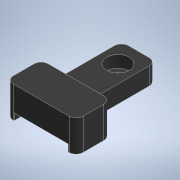
# Autodesk Inventor part: 28_Switch_Holder_Y
Saved by Autodesk Inventor 2022.2 (Build 262287010, 287A)
## iProperties
Created: 2022-05-06
Part Number: 28_Switch_Holder_Y
Material: PET-Kunststoff
Document SubType Name: Modeling
Designer: MXBD
Density: 1.541 g/cm^3
Appearance: Gummi - Schwarz
Author: MXBD
Autodesk Inventor part; units mm, degrees
ref_plane "YZ Plane" through (0, 0, 0) normal (1, 0, 0) x (0, 1, 0)
ref_plane "XZ Plane" through (0, 0, 0) normal (0, 1, 0) x (-1, 0, 0)
ref_plane "XY Plane" through (0, 0, 0) normal (0, 0, 1) x (1, 0, 0)
sketch "Skizze1" plane through (0, 0, 0) normal (0, 1, 0) x (-1, 0, 0)
  line L0 (0, -28.6) -> (0, 10.6) projected
  line L1 (-14, 0) -> (14, 0) projected
  line L2 (-10, 5) -> (10, 5)
  line L3 (10, 5) -> (10, -5)
  line L4 (10, -5) -> (-10, -5)
  line L5 (-10, -5) -> (-10, 5)
  line L6 (-10, 5) -> (10, -5) construction
  line L7 (10, 5) -> (-10, -5) construction
  line L8 (-5, -5) -> (5, -5)
  line L9 (5, -5) -> (5, -23)
  line L10 (5, -23) -> (-5, -23)
  line L11 (-5, -23) -> (-5, -5)
  line L12 (-5, -5) -> (5, -23) construction
  line L13 (5, -5) -> (-5, -23) construction
  point P0 (0, 0)
  point P1 (0, -14)
  point P2 (-5, -5)
  point P3 (5, -5)
  dimension "d0" = 20
  dimension "d1" = 10
  dimension "d2" = 10
  dimension "d3" = 18
  constraints: 24 end point, 4 midpoint, 4 parallel, 2 horizontal, 2 perpendicular, 1 collinear, 1 point on line
  measures "d0" distance of L3.end L4.end
  measures "d1" distance of L2.end L3.end
  measures "d2" distance of L9.end L10.end
  measures "d3" distance of L8.end L9.end
extrude "Extrusion1" add sketch "Skizze1" along normal blind 5
sketch "Skizze2" plane through (0, 5, 0) normal (0, 1, 0) x (1, 0, 0)
  line L0 (0, 28.6) -> (0, -10.6) projected
  line L1 (5, 23) -> (-5, 23) projected
  line L2 (-10, -5) -> (10, -5) projected
  point P0 (0, 0)
  point P1 (0, 17)
  dimension "d14" = 22
  constraints: 1 point on line
  measures "d14" distance from line of point (0, 17) L2
hole "Bohrung1" at (0, 5, -17) direction (0, -1, 0) diameter 3.4 end through all counterbore diameter 6.5 counterbore depth 3.4 clearance for "Inbusschraube ISO 4762" size "M3" standard "ISO"
sketch "Skizze3" plane through (0, 5, 0) normal (0, 1, 0) x (1, 0, 0)
  line L0 (-10, -5) -> (10, -5) projected
  line L1 (10, -5) -> (10, 5) projected
  line L2 (-10, -5) -> (10, -5)
  line L3 (10, -5) -> (10, 5)
  line L4 (10, 5) -> (-10, 5)
  line L5 (-10, 5) -> (-10, -5)
  point P0 (0, 0)
  constraints: 8 end point, 2 parallel, 1 horizontal, 1 perpendicular
extrude "Extrusion2" add sketch "Skizze3" along normal blind 2
sketch "Skizze4" plane through (0, 0, 0) normal (0, -1, 0) x (1, 0, 0)
  line L0 (-10, 5) -> (10, 5) projected
  line L1 (10, -5) -> (5, -5) projected
  line L2 (10, 5) -> (7.75, 5)
  line L3 (7.75, 5) -> (7.75, -5)
  line L4 (7.75, -5) -> (10, -5)
  line L5 (10, -5) -> (10, 5)
  point P0 (0, 0)
  dimension "d17" = 2.25
  constraints: 8 end point, 2 parallel, 1 horizontal, 1 perpendicular, 1 point on line
  measures "d17" distance of L4.end L3.end
extrude "Extrusion3" add sketch "Skizze4" along normal blind 2
mirror "Spiegeln1" about plane through (0, 0, 0) normal (1, 0, 0) of "Extrusion3"
fillet "Rundung1" radius 2 4 edges at (5, 2.5, -23) (-5, 2.5, -23) (10, 2.5, 5) (-10, 2.5, 5)
fillet "Rundung2" radius 2 2 edges at (10, 2.5, -5) (-10, 2.5, -5)
